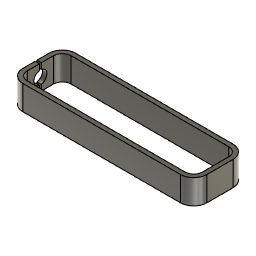
Thermistor Silicon Mold (Autodesk Fusion 360 design; units mm, degrees)
Autodesk Fusion 360 part; units mm, degrees
sketch "Base" plane through (0, 0, 0) normal (0, 0, 1) x (1, 0, 0) in component " Thermistor Silicon Mold"
  line L0 (0, 0) -> (42, 0)
  line L1 (42, 0) -> (42, 12)
  line L2 (42, 12) -> (0, 12)
  line L3 (0, 12) -> (0, 0)
  dimension "d1" = 42
  dimension "d2" = 12
  constraint horizontal L0
  constraint vertical L1
  constraint horizontal L2
  constraint vertical L3
  constraint coincident L0.start L3.end
  measures "d1" distance of L0.start L0.end
  measures "d2" distance of L0.start L2.end
extrude "Extrude1" add sketch "Base" along normal blind 5.6 in component " Thermistor Silicon Mold"
fillet "Fillet1" radius 3 4 edges at (0, 0, 2.8) (42, 0, 2.8) (42, 12, 2.8) (0, 12, 2.8) in component " Thermistor Silicon Mold"
sketch "Hollow" plane through (0, 0, 5.6) normal (0, 0, 1) x (-1, 0, 0) in component " Thermistor Silicon Mold"
  arc A0 (-3, -12) -> (0, -9) centre (-3, -9) ccw
  line L0 (0, -9) -> (0, -3)
  arc A1 (0, -3) -> (-3, 0) centre (-3, -3) ccw
  line L1 (-3, 0) -> (-39, 0)
  arc A2 (-39, 0) -> (-42, -3) centre (-39, -3) ccw
  line L2 (-42, -3) -> (-42, -9)
  arc A3 (-42, -9) -> (-39, -12) centre (-39, -9) ccw
  line L3 (-39, -12) -> (-3, -12)
  line L4 (-1, -9) -> (-1, -3)
  arc A4 (-1, -3) -> (-3, -1) centre (-3, -3) ccw
  line L5 (-3, -1) -> (-39, -1)
  arc A5 (-39, -1) -> (-41, -3) centre (-39, -3) ccw
  line L6 (-41, -3) -> (-41, -9)
  arc A6 (-41, -9) -> (-39, -11) centre (-39, -9) ccw
  line L7 (-39, -11) -> (-3, -11)
  arc A7 (-3, -11) -> (-1, -9) centre (-3, -9) ccw
  dimension "d7" = -1
extrude "Extrude2" cut sketch "Hollow" against normal up to surface (5.6 mm away) contours L4 A4 L5 A5 L6 A6 L7 A7 in component " Thermistor Silicon Mold"
sketch "Hole" plane through (0, 0, 0) normal (-1, 0, 0) x (0, -1, 0) in component " Thermistor Silicon Mold"
  line L0 (-9, 5.6) -> (-9, 0)
  line L1 (-9, 0) -> (-3, 0)
  line L2 (-3, 0) -> (-3, 5.6)
  line L3 (-3, 5.6) -> (-9, 5.6)
  line L4 (-6, 5.6) -> (-6, 0) construction
  line L5 (-9, 2.8) -> (-3, 2.8) construction
  circle A0 centre (-6, 2.8) radius 1.5
  dimension "d10" = 3
  constraint midpoint L3 L4.start
  constraint midpoint L1 L4.end
  constraint midpoint L0 L5.start
  constraint midpoint L2 L5.end
  constraint midpoint L5 A0.centre
  measures "d10" diameter of A0
extrude "Extrude3" cut sketch "Hole" against normal up to surface (1 mm away) contours A0 in component " Thermistor Silicon Mold"
sketch "Cut Through" plane through (0, 0, 0) normal (-1, 0, 0) x (0, -1, 0) in component " Thermistor Silicon Mold"
  circle A0 centre (-6, 2.8) radius 1.5
  line L0 (-9, 5.6) -> (-9, 0)
  line L1 (-9, 0) -> (-3, 0)
  line L2 (-3, 0) -> (-3, 5.6)
  line L3 (-3, 5.6) -> (-9, 5.6)
  line L4 (-6, 5.6) -> (-6, 0) construction
  line L5 (-6, 5.6) -> (-6.2, 5.6)
  line L6 (-6, 5.6) -> (-5.8, 5.6)
  line L7 (-6.2, 5.6) -> (-6.2, 0)
  line L8 (-5.8, 5.6) -> (-5.8, 0)
  line L9 (-6.2, 0) -> (-5.8, 0)
  dimension "d13" = 0.2
  dimension "d14" = 0.2
  constraint midpoint L3 L4.start
  constraint midpoint L1 L4.end
  constraint perpendicular L4 L5
  constraint perpendicular L4 L6
  constraint coincident L1 L7.end
  constraint perpendicular L1 L7
  constraint coincident L1 L8.end
  constraint perpendicular L1 L8
  measures "d13" distance of L4.start L5.end
  measures "d14" distance of L4.start L6.end
extrude "Extrude4" cut sketch "Cut Through" against normal up to surface (1 mm away) contours A0 L3 L5 L6 L7 L8 | A0 L1 L7 L8 L9 in component " Thermistor Silicon Mold"
component " Thermistor Silicon Mold" placed x (1, 0, 0) y (0, 1, 0) z (0, 0, 1) at (-1.1446, -0.9044, -0.1917)
